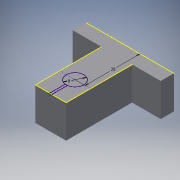
# Autodesk Inventor part: YRodClamp
Saved by Autodesk Inventor 2019 (Build 230136000, 136)
## iProperties
Created: 2019-08-21
Part Number: YRodClamp
Material: Generic
Document SubType Name: Modeling
Designer: Bruno
Density: 1 g/cm^3
Appearance: Default
Author: Bruno
Autodesk Inventor part; units mm, degrees
ref_plane "YZ Plane" through (0, 0, 0) normal (1, 0, 0) x (0, 1, 0)
ref_plane "XZ Plane" through (0, 0, 0) normal (0, 1, 0) x (-1, 0, 0)
ref_plane "XY Plane" through (0, 0, 0) normal (0, 0, 1) x (1, 0, 0)
sketch "Sketch1" plane through (0, 0, 0) normal (0, 0, 1) x (1, 0, 0)
  line L0 (-11.7577, -18.2929) -> (28.2423, -18.2929)
  line L1 (28.2423, -18.2929) -> (28.2423, -3.2929)
  line L2 (28.2423, -3.2929) -> (-11.7577, -3.2929)
  line L3 (-11.7577, -3.2929) -> (-11.7577, -18.2929)
  point P0 (0, 0)
  dimension "d0" = 40
  dimension "d1" = 15
  constraints: 8 end point, 2 parallel, 1 horizontal, 1 perpendicular
  measures "d0" distance of L0.start L0.end
  measures "d1" distance of L0.end L1.end
extrude "Extrusion1" add sketch "Sketch1" along normal blind 6
sketch "Sketch2" plane through (0, 0, 6) normal (0, 0, 1) x (1, 0, 0)
  line L0 (28.2423, -3.2929) -> (-11.7577, -3.2929) projected
  line L1 (15.2423, -3.2929) -> (15.2423, -18.2929)
  line L2 (1.2423, -3.2929) -> (1.2423, -18.2929)
  line L3 (-11.7577, -18.2929) -> (28.2423, -18.2929) projected
  line L4 (15.2423, -6.7382) -> (28.2423, -6.7382) construction
  line L5 (28.2423, -18.2929) -> (28.2423, -3.2929) projected
  line L6 (1.2423, -6.7382) -> (-11.7577, -6.7382) construction
  line L7 (-11.7577, -3.2929) -> (-11.7577, -18.2929) projected
  point P0 (0, 0)
  dimension "d4" = 14
  constraints: 10 point on line, 8 end point, 1 collinear, 1 horizontal, 1 perpendicular, 1 vertical
  measures "d4" distance between parallel lines of L2 L1
extrude "Extrusion2" add sketch "Sketch2" along normal blind 35 contours L1 L3 L2 L0
sketch "Sketch4" plane through (0, 0, 6) normal (0, 0, 1) x (1, 0, 0)
  circle A0 centre (21.7423, -10.7929) radius 2.125
  line L0 (21.7423, -10.7929) -> (21.7423, -3.2929) construction
  line L1 (21.7423, -10.7929) -> (21.7423, -18.2929) construction
  line L2 (15.2423, -18.2929) -> (28.2423, -18.2929) projected
  line L3 (21.7423, -10.7929) -> (28.2423, -10.7929) construction
  line L4 (21.7423, -10.7929) -> (15.2423, -10.7929) construction
  line L5 (15.2423, -18.2929) -> (15.2423, -3.2929) projected
  line L6 (28.2423, -3.2929) -> (15.2423, -3.2929) projected
  line L7 (28.2423, -18.2929) -> (28.2423, -3.2929) projected
  circle A1 centre (-5.2577, -10.7929) radius 2.125
  line L8 (-5.2577, -10.7929) -> (-5.2577, -3.2929) construction
  line L9 (-5.2577, -10.7929) -> (-11.7577, -10.7929) construction
  line L10 (-11.7577, -3.2929) -> (-11.7577, -18.2929) projected
  line L11 (-5.2577, -10.7929) -> (-5.2577, -18.2929) construction
  line L12 (-5.2577, -10.7929) -> (1.2423, -10.7929) construction
  line L13 (1.2423, -3.2929) -> (1.2423, -18.2929) projected
  point P0 (0, 0)
  dimension "d12" = 4.25
  dimension "d13" = 4.25
  constraints: 16 end point, 6 midpoint, 4 collinear, 3 horizontal, 3 vertical, 2 centre point
  measures "d12" diameter of A0
  measures "d13" diameter of A1
extrude "Extrusion4" cut sketch "Sketch4" against normal up to next contours A0 | A1
sketch "Sketch5" plane through (1.2423, -18.2929, 6) normal (-1, 0, 0) x (0, 0, 1)
  circle A0 centre (19, 7.5) radius 4
  line L0 (19, 7.5) -> (19, 15) construction
  line L1 (19, 7.5) -> (19, 0) construction
  line L2 (-6, 15) -> (-6, 0) projected
  line L3 (22.9686, 7) -> (35, 7)
  line L4 (22.9686, 8) -> (35, 8)
  line L5 (35, 15) -> (35, 0) projected
  line L6 (27.4068, 8) -> (27.4068, 15) construction
  line L7 (27.4068, 7) -> (27.4068, 0) construction
  line L8 (0, 0) -> (35, 0) projected
  line L9 (0, 15) -> (35, 15) projected
  line L10 (19, 7.5) -> (19, 0) construction
  line L11 (0, 0) -> (35, 0) projected
  point P0 (-6, 18.2929)
  dimension "d16" = 8
  dimension "d17" = 25
  dimension "d18" = 1
  constraints: 14 end point, 8 point on line, 4 vertical, 3 collinear, 2 horizontal, 2 point on circle, 1 centre point, 1 perpendicular
  measures "d16" diameter of A0
  measures "d17" distance between parallel lines of L2 L0
  measures "d18" distance between parallel lines of L3 L4
extrude "Extrusion5" cut sketch "Sketch5" against normal up to next
sketch "Sketch6" plane through (-11.7577, -3.2929, 0) normal (0, 1, 0) x (1, 0, 0)
  circle A0 centre (20, -35) radius 2.125
  line L0 (27, -41) -> (13, -41) projected
  line L1 (20, -35) -> (27, -35) construction
  line L2 (20, -35) -> (13, -35) construction
  line L3 (27, -6) -> (27, -41) projected
  line L4 (13, -6) -> (13, -41) projected
  point P0 (11.7577, 0)
  dimension "d21" = 4.25
  dimension "d22" = 6
  constraints: 4 end point, 2 horizontal, 2 point on line, 1 centre point, 1 collinear
  measures "d21" diameter of A0
  measures "d22" distance from line of L1.start L0
extrude "Extrusion6" cut sketch "Sketch6" against normal through all
body "Solid1"
